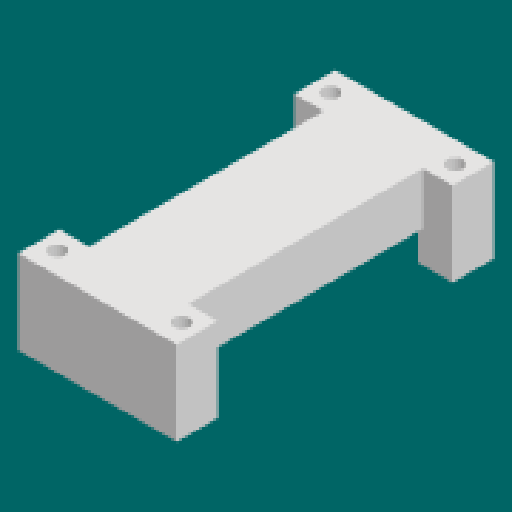
# Autodesk Inventor part: atas
Saved by Autodesk Inventor 2025.2 (Build 292293000, 293)
## iProperties
Created: 2025-04-22
Part Number: atas
Material: Generic
Document SubType Name: Modeling
Designer: ia088
Density: 1 g/cm^3
Appearance: Default
Author: ia088
Autodesk Inventor part; units mm, degrees
ref_plane "YZ Plane" through (0, 0, 0) normal (1, 0, 0) x (0, 1, 0)
ref_plane "XZ Plane" through (0, 0, 0) normal (0, 1, 0) x (-1, 0, 0)
ref_plane "XY Plane" through (0, 0, 0) normal (0, 0, 1) x (1, 0, 0)
sketch "Sketch1" plane through (0, 0, 0) normal (0, 1, 0) x (-1, 0, 0)
  line L0 (50, 100) -> (-50, 100)
  line L1 (-50, 100) -> (-50, -100)
  line L2 (-50, -100) -> (50, -100)
  line L3 (50, -100) -> (50, 100)
  line L4 (50, 100) -> (-50, -100) construction
  line L5 (-50, 100) -> (50, -100) construction
  line L6 (-47, -97) -> (47, -97)
  line L7 (47, -97) -> (47, 97)
  line L8 (47, 97) -> (-47, 97)
  line L9 (-47, 97) -> (-47, -97)
  line L10 (-47, -97) -> (47, 97) construction
  line L11 (47, -97) -> (-47, 97) construction
  line L12 (50, 100) -> (50, 77)
  line L13 (50, 77) -> (-50, 77)
  line L14 (0, 0) -> (10.1877, 0)
  line L15 (50, -77) -> (-50, -77)
  line L16 (0, 0) -> (0, -5.3943)
  line L17 (0, 100) -> (0, -100)
  line L18 (47, 97) -> (31.3333, 97)
  circle A0 centre (39.1667, 86.2777) radius 5
  line L19 (39.1667, 86.2777) -> (47, 86.2777)
  line L20 (39.1667, 86.2777) -> (31.3333, 86.2777)
  line L21 (31.3333, 86.2777) -> (31.3333, 77)
  line L22 (31.3333, 97) -> (31.3333, 86.2777)
  line L23 (0, 0) -> (-10.1877, 0)
  circle A1 centre (-39.1667, 86.2777) radius 5
  line L24 (-31.3333, 86.2777) -> (-31.3333, 77)
  line L25 (-31.3333, 97) -> (-31.3333, 86.2777)
  circle A2 centre (39.1667, -86.2777) radius 5
  line L26 (31.3333, -86.2777) -> (31.3333, -77)
  line L27 (31.3333, -97) -> (31.3333, -86.2777)
  circle A3 centre (-39.1667, -86.2777) radius 5
  line L28 (-31.3333, -86.2777) -> (-31.3333, -77)
  line L29 (-31.3333, -97) -> (-31.3333, -86.2777)
  line L30 (-31.3333, 77) -> (-31.3333, -77)
  line L31 (31.3333, 77) -> (31.3333, -77)
  line L32 (39.1667, 86.2777) -> (39.1667, -86.2777)
  line L33 (-39.1667, 86.2777) -> (-39.1667, -86.2777)
  line L34 (50, 77) -> (50, 74)
  line L35 (50, 74) -> (31.3333, 74)
  line L36 (50, -77) -> (50, -74)
  line L37 (50, -74) -> (31.3333, -74)
  line L38 (-31.3333, 77) -> (-31.3333, 74)
  line L39 (-31.3333, 74) -> (-50, 74)
  line L40 (-50, -77) -> (-50, -74)
  line L41 (-50, -74) -> (-31.3333, -74)
  dimension "d0" = 100
  dimension "d1" = 200
  dimension "d2" = 94
  dimension "d3" = 194
  dimension "d4" = 23
  dimension "d6" = 10
  dimension "d7" = 7.8333
  dimension "d8" = 7.8333
  dimension "d11" = 3
  dimension "d12" = 3
  dimension "d13" = 3
  dimension "d14" = 3
  constraints: 84 end point, 15 point on line, 15 symmetric about line, 8 perpendicular, 6 midpoint, 4 centre point, 4 horizontal, 4 parallel, 4 vertical, 3 other
  measures "d0" distance of L2.end L1.end
  measures "d1" distance of L1.end L0.end
  measures "d2" distance of L8.end L7.end
  measures "d3" distance of L7.end L6.end
  measures "d4" distance of L0.start L12.end
  measures "d6" diameter of A0
  measures "d7" distance of L19.start L19.end
  measures "d8" distance of L19.start L20.end
  measures "d11" distance of L12.end L34.end
  measures "d12" distance of L15.start L36.end
  measures "d13" distance of L24.end L38.end
  measures "d14" distance of L15.end L40.end
extrude "Extrusion1" add sketch "Sketch1" along normal blind 3 contours L3 L13 L7 L8 L17 L0 | L17 L8 L9 L13 L1 L0 | L3 L35 L7 L13 | L17 L13 L24 L25 L8 | L8 L22 L21 L13 L17 | L13 L32 A0 L19 L7 | L7 L35 L32 L13 | L13 L9 L39 L1 | L8 L7 L19 A0 L20 L22 | L25 L24 L13 L9 L8 | L17 L16 L15 L30 L13 | L13 L31 L15 L17 L16 | L3 L15 L7 L37 | L32 L35 L31 L13 | L13 L21 L20 A0 L32 | L13 L33 L39 L9 | L30 L39 L33 L13 | L3 L2 L17 L6 L7 L15 | L7 L15 L32 L37 | L41 L9 L15 L1 | L7 L6 L27 L26 L15 | L32 L15 L31 L37 | L15 L9 L6 L17 L2 L1 | L41 L33 L15 L9 | L30 L15 L33 L41 | L17 L6 L29 L28 L15 | L15 L26 L27 L6 L17 | L15 L28 L29 L6 L9
sketch "Sketch2" plane through (0, 0, 0) normal (0, -1, 0) x (1, 0, 0)
  line L0 (50, -74) -> (50, -100) projected
  line L1 (31.3333, -74) -> (50, -74) projected
  line L2 (31.3333, 74) -> (31.3333, -74) projected
  line L3 (50, 74) -> (31.3333, 74) projected
  line L4 (50, 100) -> (50, 74) projected
  line L5 (-50, 100) -> (50, 100) projected
  line L6 (-50, 74) -> (-50, 100) projected
  line L7 (-31.3333, 74) -> (-50, 74) projected
  line L8 (-31.3333, -74) -> (-31.3333, 74) projected
  line L9 (-50, -74) -> (-31.3333, -74) projected
  line L10 (-50, -100) -> (-50, -74) projected
  line L11 (50, -100) -> (-50, -100) projected
  line L12 (28.3333, -77) -> (47, -77)
  line L13 (47, -77) -> (47, -97)
  line L14 (47, -97) -> (-47, -97)
  line L15 (-47, -97) -> (-47, -77)
  line L16 (-47, -77) -> (-28.3333, -77)
  line L17 (-28.3333, -77) -> (-28.3333, 77)
  line L18 (-28.3333, 77) -> (-47, 77)
  line L19 (-47, 77) -> (-47, 97)
  line L20 (-47, 97) -> (47, 97)
  line L21 (47, 97) -> (47, 77)
  line L22 (47, 77) -> (28.3333, 77)
  line L23 (28.3333, 77) -> (28.3333, -77)
  point P0 (0, 0)
  dimension "d15" = 3
  constraints: 24 end point, 11 other
  measures "d15" distance between parallel lines of L2 L23
extrude "Extrusion2" add sketch "Sketch2" along normal blind 30
sketch "Sketch3" plane through (0, -30, 0) normal (0, -1, 0) x (1, 0, 0)
  line L0 (31.3333, 74) -> (50, 74) projected
  line L1 (50, 74) -> (50, 100) projected
  line L2 (50, 100) -> (-50, 100) projected
  line L3 (-50, 100) -> (-50, 74) projected
  line L4 (-50, 74) -> (-31.3333, 74) projected
  line L5 (-31.3333, -74) -> (-50, -74) projected
  line L6 (-50, -74) -> (-50, -100) projected
  line L7 (-50, -100) -> (50, -100) projected
  line L8 (50, -100) -> (50, -74) projected
  line L9 (50, -74) -> (31.3333, -74) projected
  line L10 (28.3333, -77) -> (47, -77) projected
  line L11 (47, -77) -> (47, -97) projected
  line L12 (47, -97) -> (-47, -97) projected
  line L13 (-47, -97) -> (-47, -77) projected
  line L14 (-47, -77) -> (-28.3333, -77) projected
  line L15 (-28.3333, -77) -> (-28.3333, 77) projected
  line L16 (-28.3333, 77) -> (-47, 77) projected
  line L17 (-47, 77) -> (-47, 97) projected
  line L18 (-47, 97) -> (47, 97) projected
  line L19 (47, 97) -> (47, 77) projected
  line L20 (47, 77) -> (28.3333, 77) projected
  line L21 (28.3333, 77) -> (28.3333, -77) projected
  line L22 (31.3333, 74) -> (-50, 74)
  line L23 (31.3333, -74) -> (-50, -74)
  point P0 (0, 0)
  point P1 (28.3333, -74)
  point P2 (-28.3333, -74)
  point P3 (-28.3333, 74)
  point P4 (28.3333, 74)
  constraints: 4 end point, 2 collinear
extrude "Extrusion3" add sketch "Sketch3" along normal blind 20 contours L22 L21 L20 L19 L18 L17 L16 L15 L4 L3 L2 L1 L0 | L23 L9 L8 L7 L6 L5 L15 L14 L13 L12 L11 L10 L21
sketch "Sketch4" plane through (0, 0, 0) normal (0, -1, 0) x (1, 0, 0)
  line L0 (28.3333, 77) -> (47, 77) projected
  line L1 (47, 77) -> (47, 97) projected
  line L2 (47, 97) -> (-47, 97) projected
  line L3 (-47, 97) -> (-47, 77) projected
  line L4 (-47, 77) -> (-28.3333, 77) projected
  line L5 (-28.3333, -77) -> (-47, -77) projected
  line L6 (-47, -77) -> (-47, -97) projected
  line L7 (-47, -97) -> (47, -97) projected
  line L8 (47, -97) -> (47, -77) projected
  line L9 (47, -77) -> (28.3333, -77) projected
  circle A0 centre (39.1667, -86.2777) radius 5 projected
  circle A1 centre (39.1667, 86.2777) radius 5 projected
  circle A2 centre (-39.1667, -86.2777) radius 5 projected
  circle A3 centre (-39.1667, 86.2777) radius 5 projected
  line L10 (28.3333, 77) -> (28.3333, 97)
  line L11 (-28.3333, 77) -> (-28.3333, 97)
  line L12 (-28.3333, -77) -> (-28.3333, -97)
  line L13 (28.3333, -77) -> (28.3333, -97)
  point P0 (0, 0)
  constraints: 8 end point, 6 point on line, 1 parallel, 1 perpendicular
extrude "Extrusion4" add sketch "Sketch4" along normal up to surface (50 mm away)
body "Solid1"
